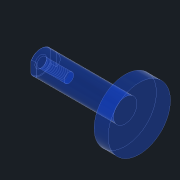
# Autodesk Inventor part: SDA-32x2525_r
Saved by Autodesk Inventor 2022 (Build 260153000, 153)
## iProperties
Category: PARTsolutions
Company: AIRTAC
Created: 2022-09-20
Part Number: SDA-32x2525_r
Material: Generic
Catalog Web Link: www.cadenas.de
Description: SDA SSA STA  Series - Rod-Rod
Vendor: AIRTAC
Document SubType Name: Modeling
Designer: psAdmin
Manufacturer: AIRTAC
Mass: 10.3353 g
Surface Area: 41.6163 cm^2
Volume: 10.3353 cm^3
Density: 1 g/cm^3
Appearance: PSOLRGB-175-175-175
PSOL_IDENT_0: {$CADENAS_DATA/23d-libs/airtac/pneumatic_equipment/cylinders/compact_cylinder/sda_series/parts/sda_s
PSOL_IDENT_1: sa_sta_rod.prj},227 {VTYP=3D},{NB=SDA-32x2525_r},{LINA=SDA-32x25},{NN=SDA SSA STA  Series - Rod},{DA
PSOL_IDENT_2: TE=27.08.2021 03:42:35},{GEOMDATE=16.04.2020 11:33:42},{VERSION=},{LINEID=50},{WBVAR=TYPE,STROKE,STR
PSOL_IDENT_3: OKE1,MAGNET,RTYPE},{WBNUMERIC=STROKE,STROKE1}  {NB=SDA-32x2525_r},{LINA=SDA-32x25},{KT=DUMMY},{BORE=
PSOL_IDENT_4: 32},{TYPE=SDA},{STROKE=25},{STROKE1=25},{MAGNET=},{RTYPE=},{ST1=5,10,15,20,25,30,35,40,45,50,55,60,6
PSOL_IDENT_5: 5,70,75,80,85,90,100,110,120,130,[5:100]},{ORDER=SDA-32x25},{A=31.5},{B1=7.0},{B2=25.000},{C=24.5},{
PSOL_IDENT_6: D=50.0},{E=12},{F=4},{G=3.0},{H=15.000},{K1=M6×1.0},{K11=6.000},{K12=1.000},{K21=10.000},{K2=M10×1.2
PSOL_IDENT_7: 5},{K22=1.250},{L=22.0},{M=3},{N1=9.0},{N2=9.0},{O=PT1/8},{P1=4.6},{P2=M6×1.0},{P3=16},{P4=5.5},{P5=
PSOL_IDENT_8: 8.2},{R=6},{S=44},{T1=34.0},{U=2.0},{V=12},{W=10},{X=18.3},{Y=15},{TYPE1='SDA', 'SDA Type', 'SSA', '
PSOL_IDENT_9: SSA Type', 'STA', 'STA Type'},{R1=3.000},{R2=0.100},{ST2=25}
NB: SDA-32x2525_r
NN: SDA SSA STA  Series - Rod
NT: Rod
NBSYN: $ORDER.$STROKE._r
LINA: SDA-32x25
CATALOG: AirTAC
BORE: 32
TYPE: SDA Type
STROKE: 25
STROKE1: 25
MAGNET: Without cushion
RTYPE: Female thread
B1: 7
B2: 25
D: 50
F: 4
G: 3
H: 15
K1: M6×1.0
K11: 6
K12: 1
K21: 10
K2: M10×1.25
K22: 1.25
L: 22
M: 3
O: PT1/8
P1: 4.6
P2: M6×1.0
P3: 16
P4: 5.5
P5: 8.2
R: 6
S: 44
T1: 34
U: 2
V: 12
W: 10
X: 18.3
Y: 15
R1: 3
R2: 0.1
SUPPLIER: AIRTAC
ARTICLENO: SDA-32x2525_r
BOMINFO: SDA-32x25
CREATOR: CADENAS GmbH
Title: SDA-32x25
Author: Cadenas PARTsolutions
Comments: Rod
Autodesk Inventor part; units mm, degrees
sketch "Sketch_12" plane through (0, 0, 0) normal (0, 0, 1) x (1, 0, 0)
  line L0 (0, 0) -> (-7, 0)
  line L1 (-7, 0) -> (-7, 5.75)
  line L2 (-7, 5.75) -> (-6.75, 6)
  line L3 (-6.75, 6) -> (0, 6)
  line L4 (0, 6) -> (0, 0)
  line L5 (0, 0) -> (-7, 0)
  constraints: 12 end point
revolve "Revolution1" add sketch "Sketch_12" angle 360 about axis through (0, 0, 0) along (1, 0, 0)
sketch "Sketch_16" plane through (0, 0, 0) normal (0, 0, 1) x (1, 0, 0)
  line L0 (43.5, 0) -> (0, 0)
  line L1 (0, 0) -> (0, 6)
  line L2 (0, 6) -> (36.3, 6)
  line L3 (36.3, 6) -> (36.3, 15.95)
  line L4 (36.3, 15.95) -> (43.5, 15.95)
  line L5 (43.5, 15.95) -> (43.5, 0)
  line L6 (43.5, 0) -> (0, 0)
  constraints: 14 end point
revolve "Revolution2" add sketch "Sketch_16" angle 360 about axis through (43.5, 0, 0) along (1, 0, 0)
sketch "Sketch_13" plane through (0, 0, 0) normal (0, 1, 0) x (-1, 0, 0)
  line L0 (17, -10) -> (17, 10)
  line L1 (17, 10) -> (-1, 10)
  line L2 (-1, 10) -> (4, 5)
  line L3 (4, 5) -> (7, 5)
  line L4 (7, 5) -> (7, -5)
  line L5 (7, -5) -> (4, -5)
  line L6 (4, -5) -> (-1, -10)
  line L7 (-1, -10) -> (17, -10)
  constraints: 16 end point
extrude "Extrusion1" cut sketch "Sketch_13" along normal mid plane 20
sketch "Sketch4" plane through (-7, -2.8395, 5) normal (-1, 0, 0) x (0, 0, 1)
  point P0 (-5, 2.8395)
hole "Hole1" at (-7, 0, 0) direction (1, 0, 0) diameter 4.917 depth 14.4 tip angle 120 countersink diameter 6 countersink angle 90 thread size "M6x1" class "6H" standard "ISO Metric profile"
ref_plane "for_body_XY" through (0, 0, 0) normal (1, 0, 0) x (0, 0, -1)
ref_plane "for_body_YZ" through (0, 0, 0) normal (0, 0, -1) x (0, 1, 0)
ref_plane "for_body_ZX" through (0, 0, 0) normal (0, 1, 0) x (1, 0, 0)
ref_plane "for_nut_XY" through (-17.5, 0, 0) normal (-1, 0, 0) x (0, 0, -1)
ref_plane "for_nut_YZ" through (-17.5, 0, 0) normal (0, 0, -1) x (0, -1, 0)
ref_plane "for_nut_ZX" through (-17.5, 0, 0) normal (0, -1, 0) x (-1, 0, 0)
body "Solid1"
